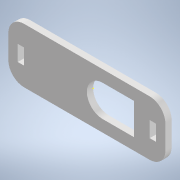
# Autodesk Inventor part: top
Saved by Autodesk Inventor 2022 (Build 260153000, 153)
## iProperties
Created: 2025-06-24
Part Number: top
Material: Типовые
Document SubType Name: Modeling
Designer: korsh524
Density: 1 g/cm^3
Appearance: По умолчанию
Author: korsh524
Autodesk Inventor part; units mm, degrees
ref_plane "YZ Plane" through (0, 0, 0) normal (1, 0, 0) x (0, 1, 0)
ref_plane "XZ Plane" through (0, 0, 0) normal (0, 1, 0) x (-1, 0, 0)
ref_plane "XY Plane" through (0, 0, 0) normal (0, 0, 1) x (1, 0, 0)
sketch "Эскиз1" plane through (0, 0, 0) normal (0, 0, 1) x (1, 0, 0)
  line L0 (40, -17.5) -> (22.4906, -17.5) projected
  arc A0 (40, -17.5) -> (50, -7.5) centre (40, -7.5) ccw projected
  line L1 (50, 7.5) -> (50, -7.5) projected
  arc A1 (50, 7.5) -> (40, 17.5) centre (40, 7.5) ccw projected
  line L2 (22.4906, 17.5) -> (40, 17.5) projected
  arc A2 (22.4906, 17.5) -> (53.3569, 60.2081) centre (-76.5583, 121.5932) ccw projected
  arc A3 (53.3569, 60.2081) -> (49.04, 63.7734) centre (57.3118, 69.3928) ccw projected
  arc A4 (49.04, 63.7734) -> (8.22, 17.5) centre (133.8701, -52.2004) ccw projected
  line L3 (-8.22, 17.5) -> (8.22, 17.5) projected
  arc A5 (-8.22, 17.5) -> (-49.04, 63.7734) centre (-133.8701, -52.2004) ccw projected
  arc A6 (-49.04, 63.7734) -> (-53.3569, 60.2081) centre (-57.3118, 69.3928) ccw projected
  arc A7 (-53.3569, 60.2081) -> (-22.4906, 17.5) centre (76.5583, 121.5932) ccw projected
  line L4 (-40, 17.5) -> (-22.4906, 17.5) projected
  arc A8 (-40, 17.5) -> (-50, 7.5) centre (-40, 7.5) ccw projected
  line L5 (-50, -7.5) -> (-50, 7.5) projected
  arc A9 (-50, -7.5) -> (-40, -17.5) centre (-40, -7.5) ccw projected
  line L6 (-22.4906, -17.5) -> (-40, -17.5) projected
  arc A10 (-22.4906, -17.5) -> (-53.3569, -60.2081) centre (76.5583, -121.5932) ccw projected
  arc A11 (-53.3569, -60.2081) -> (-49.04, -63.7734) centre (-57.3118, -69.3928) ccw projected
  arc A12 (-49.04, -63.7734) -> (-8.22, -17.5) centre (-133.8701, 52.2004) ccw projected
  line L7 (8.22, -17.5) -> (-8.22, -17.5) projected
  arc A13 (8.22, -17.5) -> (49.04, -63.7734) centre (133.8701, 52.2004) ccw projected
  arc A14 (49.04, -63.7734) -> (53.3569, -60.2081) centre (57.3118, -69.3928) ccw projected
  arc A15 (53.3569, -60.2081) -> (22.4906, -17.5) centre (-76.5583, -121.5932) ccw projected
  line L8 (22.4906, 17.5) -> (-22.4906, 17.5)
  line L9 (-22.4906, -17.5) -> (22.4906, -17.5)
  line L10 (25, 12.5) -> (25, 8.5) projected
  line L11 (25, 8.5) -> (15, 8.5) projected
  line L12 (15, 8.5) -> (15, 12.5) projected
  line L13 (15, 12.5) -> (25, 12.5) projected
  line L14 (-15, -8.5) -> (-15, -12.5) projected
  line L15 (-15, -12.5) -> (-25, -12.5) projected
  line L16 (-25, -12.5) -> (-25, -8.5) projected
  line L17 (-25, -8.5) -> (-15, -8.5) projected
  line L18 (25, -12.5) -> (15, -12.5) projected
  line L19 (15, -12.5) -> (15, -8.5) projected
  line L20 (15, -8.5) -> (25, -8.5) projected
  line L21 (25, -8.5) -> (25, -12.5) projected
  line L22 (-15, 8.5) -> (-25, 8.5) projected
  line L23 (-25, 8.5) -> (-25, 12.5) projected
  line L24 (-25, 12.5) -> (-15, 12.5) projected
  line L25 (-15, 12.5) -> (-15, 8.5) projected
  point P0 (0, 0)
  point P1 (8.22, 17.5)
  point P2 (-8.22, -17.5)
  constraints: 4 end point, 1 collinear, 1 horizontal
extrude "Выдавливание1" add sketch "Эскиз1" along normal blind 4 contours L0 L9 L7 L6 A9 L5 A8 L4 L8 L3 L2 A1 L1 A0 | L10 L11 L12 L13 | L14 L15 L16 L17 | L18 L19 L20 L21 | L22 L23 L24 L25
sketch "Эскиз3" plane through (0, 0, 0) normal (0, 0, -1) x (-1, 0, 0)
  point P0 (0, 0)
sketch "Эскиз4" plane through (0, 0, 0) normal (0, 0, -1) x (-1, 0, 0)
  point P0 (0, 0)
sketch "Эскиз5" plane through (0, 0, 0) normal (0, 0, -1) x (-1, 0, 0)
  line L0 (44, 4.453) -> (44, -5.547) projected
  line L1 (40, -5.547) -> (40, 4.453) projected
  line L2 (40, 4.453) -> (44, 4.453) projected
  line L3 (44, -5.547) -> (40, -5.547) projected
  line L4 (-44, -5.547) -> (-44, 4.453) projected
  line L5 (-40, 4.453) -> (-40, -5.547) projected
  line L6 (-44, 4.453) -> (-40, 4.453) projected
  line L7 (-40, -5.547) -> (-44, -5.547) projected
  line L8 (-10, 10) -> (-30, 10)
  line L9 (-30, 10) -> (-30, -10)
  line L10 (-30, -10) -> (-10, -10)
  line L11 (0, 0) -> (0, 0)
  arc A0 (0, 0) -> (-10, 10) centre (-10, 0) ccw
  arc A1 (-10, -10) -> (0, 0) centre (-10, 0) ccw
  point P0 (0, 0)
  point P1 (0, 10)
  dimension "d4" = 10
  dimension "d5" = 10
  dimension "d6" = 30
  dimension "d7" = 10
  dimension "d8" = 10
  dimension "d9" = 30
  constraints: 8 end point, 4 point on circle, 4 tangent, 2 centre point, 2 parallel, 2 point on line, 1 horizontal, 1 perpendicular
  measures "d4" distance from line of L10 point (0, 0)
  measures "d5" distance from line of L8 point (0, 0)
  measures "d6" distance of point (0, 10) L8.end
  measures "d7" radius of A0
  measures "d8" radius of A1
  measures "d9" distance from line of L9 point (0, 0)
extrude "Выдавливание3" cut sketch "Эскиз5" against normal blind 4
sketch "Эскиз6" plane through (0, 0, 0) normal (0, 0, -1) x (-1, 0, 0)
  point P0 (0, 0)
